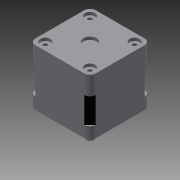
# Autodesk Inventor part: NEMA17Stepper
Saved by Autodesk Inventor 2013 (Build 170138000, 138)
## iProperties
Created: 2015-01-14
Part Number: NEMA17Stepper
Material: Generic
Document SubType Name: Modeling
Designer: dzban
Density: 1 g/cm^3
Author: dzban
Autodesk Inventor part; units mm, degrees
ref_plane "YZ Plane" through (0, 0, 0) normal (1, 0, 0) x (0, 1, 0)
ref_plane "XZ Plane" through (0, 0, 0) normal (0, 1, 0) x (-1, 0, 0)
ref_plane "XY Plane" through (0, 0, 0) normal (0, 0, 1) x (1, 0, 0)
sketch "Sketch1" plane through (0, 0, 0) normal (0, 0, 1) x (1, 0, 0)
  circle A0 centre (21, 21) radius 11
  circle A1 centre (36.5, 5.5) radius 1.5
  circle A2 centre (5.5, 36.5) radius 1.5
  circle A3 centre (5.5, 5.5) radius 1.5
  circle A4 centre (36.5, 36.5) radius 1.5
  line L0 (42, 4) -> (42, 38)
  arc A5 (42, 38) -> (38, 42) centre (38, 38) ccw
  line L1 (38, 42) -> (4, 42)
  arc A6 (4, 42) -> (0, 38) centre (4, 38) ccw
  line L2 (0, 38) -> (0, 4)
  arc A7 (0, 4) -> (4, 0) centre (4, 4) ccw
  line L3 (4, 0) -> (38, 0)
  arc A8 (38, 0) -> (42, 4) centre (38, 4) ccw
  point P0 (0, 0)
  point P1 (0, 0)
  constraints: 9 centre point, 8 end point, 8 point on circle
extrude "Extrusion1" add sketch "Sketch1" along normal blind 8 contours A0 | A8 L3 A7 L2 A6 L1 A5 L0
sketch "Sketch2" plane through (0, 0, 8) normal (0, 0, 1) x (1, 0, 0)
  circle A0 centre (36.5, 36.5) radius 1.5 projected
  circle A1 centre (5.5, 5.5) radius 1.5 projected
  circle A2 centre (5.5, 36.5) radius 1.5 projected
  circle A3 centre (36.5, 5.5) radius 1.5 projected
  line L0 (42, 4) -> (42, 38) projected
  arc A4 (42, 38) -> (38, 42) centre (38, 38) ccw projected
  line L1 (38, 42) -> (4, 42) projected
  arc A5 (4, 42) -> (0, 38) centre (4, 38) ccw projected
  line L2 (0, 38) -> (0, 4) projected
  line L3 (4, 0) -> (38, 0) projected
  arc A6 (38, 0) -> (42, 4) centre (38, 4) ccw projected
  line L4 (0, 38) -> (4, 42)
  line L5 (0, 4) -> (4, 0)
  line L6 (38, 0) -> (42, 4)
  line L7 (42, 38) -> (38, 42)
  point P0 (0, 0)
  constraints: 8 end point, 3 point on circle
extrude "Extrusion2" add sketch "Sketch2" along normal blind 18 contours L6 L3 L5 L2 L4 L1 L7 L0
sketch "Sketch3" plane through (0, 0, 26) normal (0, 0, 1) x (1, 0, 0)
  circle A0 centre (36.5, 5.5) radius 1.5 projected
  circle A1 centre (5.5, 36.5) radius 1.5 projected
  circle A2 centre (5.5, 5.5) radius 1.5 projected
  circle A3 centre (36.5, 36.5) radius 1.5 projected
  line L0 (4, 42) -> (0, 38) projected
  line L1 (0, 38) -> (0, 4) projected
  line L2 (0, 4) -> (4, 0) projected
  line L3 (4, 0) -> (38, 0) projected
  line L4 (38, 0) -> (42, 4) projected
  line L5 (42, 4) -> (42, 38) projected
  line L6 (42, 38) -> (38, 42) projected
  line L7 (38, 42) -> (4, 42) projected
  line L8 (0, 38) -> (4, 42) projected
  arc A4 (4, 42) -> (0, 38) centre (4, 38) ccw projected
  line L9 (38, 42) -> (42, 38) projected
  arc A5 (42, 38) -> (38, 42) centre (38, 38) ccw projected
  line L10 (42, 4) -> (38, 0) projected
  arc A6 (38, 0) -> (42, 4) centre (38, 4) ccw projected
  line L11 (4, 0) -> (0, 4) projected
  arc A7 (0, 4) -> (4, 0) centre (4, 4) ccw projected
  point P0 (0, 0)
extrude "Extrusion3" add sketch "Sketch3" along normal blind 13
sketch "Sketch4" plane through (0, 0, 39) normal (0, 0, 1) x (1, 0, 0)
  circle A0 centre (36.5, 36.5) radius 1.5 projected
  circle A1 centre (5.5, 5.5) radius 1.5 projected
  circle A2 centre (5.5, 36.5) radius 1.5 projected
  circle A3 centre (36.5, 5.5) radius 1.5 projected
  circle A4 centre (5.5, 36.5) radius 3.5
  circle A5 centre (5.5, 5.5) radius 3.5
  circle A6 centre (36.5, 5.5) radius 3.5
  circle A7 centre (36.5, 36.5) radius 3.5
  circle A8 centre (21, 21) radius 4.5
  point P0 (0, 0)
  dimension "d6" = 7
  dimension "d8" = 7
  dimension "d9" = 7
  dimension "d10" = 7
  dimension "d22" = 9
  dimension "d23" = 15.5
  dimension "d24" = 15.5
  constraints: 5 centre point, 4 coincident
  measures "d6" diameter of A4
  measures "d8" diameter of A7
  measures "d9" diameter of A6
  measures "d10" diameter of A5
  measures "d22" diameter of A8
  measures "d23" horizontal distance of A2.centre A8.centre
  measures "d24" horizontal distance of A0.centre A8.centre
extrude "Extrusion4" cut sketch "Sketch4" against normal blind 2
sketch "Sketch5" plane through (0, 0, 0) normal (0, 0, -1) x (-1, 0, 0)
  circle A0 centre (-36.5, 36.5) radius 1.5 projected
  circle A1 centre (-5.5, 36.5) radius 1.5 projected
  circle A2 centre (-21, 21) radius 11
  point P0 (0, 0)
  dimension "d13" = 15.5
  dimension "d14" = 15.5
  dimension "d15" = 22
  constraints: 1 centre point
  measures "d13" horizontal distance of A0.centre A2.centre
  measures "d14" horizontal distance of A1.centre A2.centre
  measures "d15" diameter of A2
extrude "Extrusion5" add sketch "Sketch5" along normal blind 2 contours A2
sketch "Sketch6" plane through (21, 21, -2) normal (0, 0, -1) x (-1, 0, 0)
  circle A0 centre (0, 0) radius 11 projected
  circle A1 centre (0, 0) radius 2.5
  point P0 (21, -21)
  dimension "d18" = 5
  constraints: 1 centre point, 1 coincident
  measures "d18" diameter of A1
extrude "Extrusion6" add sketch "Sketch6" along normal blind 17 contours A1
body "Solid1"
